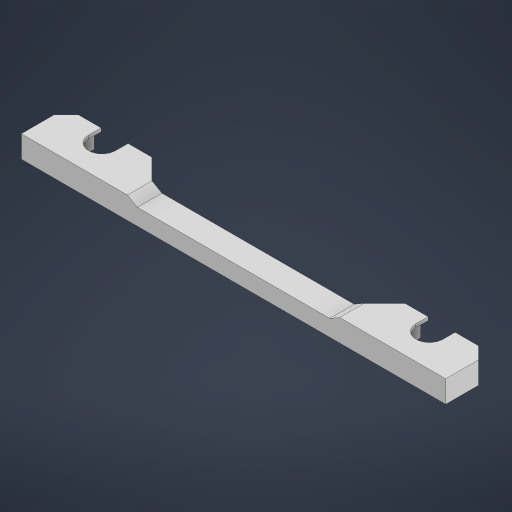
# Autodesk Inventor part: miniboard nutt holder
Saved by Autodesk Inventor 2024 (Build 280153000, 153)
## iProperties
Created: 2024-03-17
Part Number: miniboard nutt holder
Material: Všeobecné
Document SubType Name: Modeling
Designer: Simak
Density: 1 g/cm^3
Appearance: Výchozí
Author: Simak
Autodesk Inventor part; units mm, degrees
ref_plane "YZ Plane" through (0, 0, 0) normal (1, 0, 0) x (0, 1, 0)
ref_plane "XZ Plane" through (0, 0, 0) normal (0, 1, 0) x (-1, 0, 0)
ref_plane "XY Plane" through (0, 0, 0) normal (0, 0, 1) x (1, 0, 0)
sketch "Náčrt1" plane through (0, 0, 0) normal (0, 1, 0) x (-1, 0, 0)
  line L0 (14, -2) -> (10.9978, 1.0022)
  line L1 (10.9978, 1.0022) -> (-10.9978, 1.0022)
  line L2 (-10.9978, 1.0022) -> (-14, -2)
  line L3 (-14, -2) -> (-26, -2)
  line L4 (-26, -2) -> (-26, 2)
  line L5 (-26, 2) -> (26, 2)
  line L6 (26, 2) -> (26, -2)
  line L7 (26, -2) -> (14, -2)
  line L8 (20, 1.0022) -> (22.6, -0.4989)
  line L9 (22.6, -0.4989) -> (22.6, -3.5011)
  line L10 (22.6, -3.5011) -> (20, -5.0022)
  line L11 (20, -5.0022) -> (17.4, -3.5011)
  line L12 (17.4, -3.5011) -> (17.4, -0.4989)
  line L13 (17.4, -0.4989) -> (20, 1.0022)
  line L14 (-20, 1.0022) -> (-17.4, -0.4989)
  line L15 (-17.4, -0.4989) -> (-17.4, -3.5011)
  line L16 (-17.4, -3.5011) -> (-20, -5.0022)
  line L17 (-20, -5.0022) -> (-22.6, -3.5011)
  line L18 (-22.6, -3.5011) -> (-22.6, -0.4989)
  line L19 (-22.6, -0.4989) -> (-20, 1.0022)
  line L20 (26, 2) -> (0, 0) construction
  line L21 (0, 0) -> (-26, 2) construction
  line L22 (26, -2) -> (0, 0) construction
  line L23 (-17.4, -3.5011) -> (-15.5011, -3.5011)
  line L24 (-15.5011, -3.5011) -> (-14, -2)
  line L25 (17.4, -3.5011) -> (15.5011, -3.5011)
  line L26 (15.5011, -3.5011) -> (14, -2)
  line L27 (-22.6, -3.5011) -> (-24.4989, -3.5011)
  line L28 (-24.4989, -3.5011) -> (-26, -2)
  line L29 (22.6, -3.5011) -> (24.4989, -3.5011)
  line L30 (24.4989, -3.5011) -> (26, -2)
  line L31 (-13, -1) -> (13, -1)
  line L32 (-22.6, -0.4989) -> (-22.6, -0.2989)
  line L33 (-22.6, -0.2989) -> (-20, 1.2022)
  line L34 (-20, 1.2022) -> (-17.4, -0.2989)
  line L35 (-17.4, -0.2989) -> (-17.4, -0.4989)
  line L36 (17.4, -0.4989) -> (17.4, -0.2989)
  line L37 (17.4, -0.2989) -> (20, 1.2022)
  line L38 (20, 1.2022) -> (22.6, -0.2989)
  line L39 (22.6, -0.2989) -> (22.6, -0.4989)
  point P0 (20, -2)
  point P1 (-20, -2)
  dimension "d0" = 5.2
  dimension "d1" = 40
  dimension "d4" = 4
  dimension "d6" = 45
  dimension "d7" = 1
  dimension "d8" = 52
  dimension "d19" = 0.2
  dimension "d20" = 0.2
  constraints: 80 end point, 14 equal length, 8 horizontal, 7 vertical, 3 point on line, 2 collinear, 2 midpoint, 2 parallel, 26 other
  measures "d0" distance between parallel lines of L12 L9
  measures "d1" distance of point (20, -2) point (-20, -2)
  measures "d4" distance between parallel lines of L5 L3
  measures "d6" angle of L7 L30
  measures "d7" distance between parallel lines of L31 L3
  measures "d8" distance between parallel lines of L4 L6
  measures "d19" distance of L34.end L14.end
  measures "d20" distance of L38.end L8.end
extrude "Vysunutí1" add sketch "Náčrt1" along normal blind 2.7 contours L0 L1 L2 L3 L15 L35 L34 L33 L32 L18 L4 L5 L6 L7 L9 L39 L38 L37 L36 L12 | L7 L12 L25 L26 | L31 L2 L1 L0 | L7 L30 L29 L9 | L24 L23 L15 L3 | L18 L27 L28 L3
sketch "Náčrt2" plane through (0, 2.7, 0) normal (0, 1, 0) x (1, 0, 0)
  line L0 (-13, 1) -> (-15.5011, 3.5011) projected
  line L1 (-15.5011, 3.5011) -> (-17.4, 3.5011) projected
  line L2 (-17.4, 3.5011) -> (-17.4, 0.2989) projected
  line L3 (-22.6, 0.2989) -> (-22.6, 3.5011) projected
  line L4 (-22.6, 3.5011) -> (-24.4989, 3.5011) projected
  line L5 (-24.4989, 3.5011) -> (-26, 2) projected
  line L6 (-26, 2) -> (-26, -2) projected
  line L7 (-26, -2) -> (26, -2) projected
  line L8 (26, -2) -> (26, 2) projected
  line L9 (26, 2) -> (24.4989, 3.5011) projected
  line L10 (24.4989, 3.5011) -> (22.6, 3.5011) projected
  line L11 (22.6, 3.5011) -> (22.6, 0.2989) projected
  line L12 (17.4, 0.2989) -> (17.4, 3.5011) projected
  line L13 (17.4, 3.5011) -> (15.5011, 3.5011) projected
  line L14 (15.5011, 3.5011) -> (13, 1) projected
  line L15 (13, 1) -> (-13, 1) projected
  circle A0 centre (-20.075, 1.9567) radius 1.65
  circle A1 centre (20, 2) radius 1.65
  line L16 (-22.75, 0.4123) -> (-20.075, 1.9567) construction
  line L17 (-20.075, 1.9567) -> (-17.4, 0.4123) construction
  line L18 (-20.075, 1.9567) -> (-20.075, -1.1321) construction
  line L19 (20, 2) -> (22.675, 0.4556) construction
  line L20 (20, -1.0888) -> (20, 2) construction
  line L21 (17.325, 0.4556) -> (20, 2) construction
  line L22 (-22.6, 3.5011) -> (-17.4, 3.5011)
  line L23 (22.6, 3.5011) -> (17.4, 3.5011)
  line L24 (18.35, 2) -> (18.35, 3.5011)
  line L25 (21.65, 2) -> (21.65, 3.5011)
  line L26 (-18.425, 1.9567) -> (-18.425, 3.5011)
  line L27 (-21.725, 1.9567) -> (-21.725, 3.5011)
  line L28 (-17.4, 0.2989) -> (-20, -1.2022) projected
  line L29 (-20, -1.2022) -> (-22.6, 0.2989) projected
  line L30 (22.6, 0.2989) -> (20, -1.2022) projected
  line L31 (20, -1.2022) -> (17.4, 0.2989) projected
  point P0 (0, 0)
  point P1 (19.315, 3.5011)
  point P2 (20.685, 3.5011)
  point P3 (-20.6558, 3.5011)
  point P4 (-19.4942, 3.5011)
  dimension "d11" = 3.3
  constraints: 24 end point, 7 equal length, 4 perpendicular, 4 point on circle, 4 point on line, 4 tangent, 2 centre point, 1 equal radius, 1 horizontal, 1 vertical
  measures "d11" diameter of A0
extrude "Vysunutí2" add sketch "Náčrt2" against normal blind 0.4 contours L2 L28 L29 L3 L22 L27 A0 L26 | L23 L24 A1 L25 L11 L30 L31 L12
sketch "Náčrt3" plane through (13, 0, -1) normal (0, 0, -1) x (-1, 0, 0)
  line L0 (0, 0) -> (26, 0) projected
  line L1 (26, 0) -> (26, 2.7) projected
  line L2 (0, 2.7) -> (26, 2.7) projected
  line L3 (0, 0) -> (0, 2.7) projected
  line L4 (0, 2.7) -> (1.2124, 2)
  line L5 (1.2124, 2) -> (24.7876, 2)
  line L6 (24.7876, 2) -> (26, 2.7)
  point P0 (13, 0)
  dimension "d14" = 2
  dimension "d16" = 60
  constraints: 6 end point, 1 equal length, 1 horizontal
  measures "d14" distance between parallel lines of L0 L5
  measures "d16" angle of L3 L4
extrude "Vysunutí3" cut sketch "Náčrt3" against normal through all contours L2 L6 L5 L4
